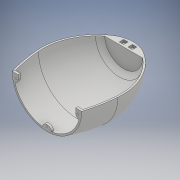
# Autodesk Inventor part: learnbotBack
Saved by Autodesk Inventor 2017 (Build 210142000, 142)
## iProperties
Part Number: learnbotBack
Material: Genérico
Document SubType Name: Modeling
Designer: rober
Density: 1 g/cm^3
Appearance: Valor por defecto
Author: rober
Autodesk Inventor part; units mm, degrees
ref_plane "YZ Plane" through (0, 0, 0) normal (1, 0, 0) x (0, 1, 0)
ref_plane "XZ Plane" through (0, 0, 0) normal (0, 1, 0) x (-1, 0, 0)
ref_plane "XY Plane" through (0, 0, 0) normal (0, 0, 1) x (1, 0, 0)
sketch "Boceto1" plane through (0, 0, 0) normal (0, 0, 1) x (1, 0, 0)
  arc A0 (-1.3629, 5.5333) -> (-0.3139, 0) centre (24.2256, 7.518) ccw
  arc A1 (-1.0638, 5.5565) -> (0, 0) centre (24.2256, 7.518) ccw
  arc A2 (3.3612, 14.9282) -> (1.4714, 13.4053) centre (8.9925, 6.0064) ccw
  arc A3 (3.5214, 14.6745) -> (1.6853, 13.1949) centre (8.9925, 6.0064) ccw
  arc A4 (6.03, 15.7) -> (3.3612, 14.9282) centre (6.03, 10.7) ccw
  arc A5 (6.03, 15.4) -> (3.5214, 14.6745) centre (6.03, 10.7) ccw
  arc A6 (1.4714, 13.4053) -> (-1.3629, 5.5333) centre (8.6002, 6.3924) ccw
  arc A7 (1.6853, 13.1949) -> (-1.0617, 5.5333) centre (8.6002, 6.3924) ccw
  line L0 (6.03, 15.4) -> (6.03, 15.7)
  line L1 (-0.3139, 0) -> (0, 0)
  line L2 (0, 0) -> (-0.3139, 0)
  line L3 (-1.0617, 5.5333) -> (-1.3629, 5.5333)
  arc A8 (-1.0617, 5.5333) -> (0, 0) centre (24.2008, 7.5121) ccw
  arc A9 (-1.3629, 5.5333) -> (-0.3139, 0) centre (24.2256, 7.518) ccw
  line L4 (6.03, 15.7) -> (6.03, 15.4)
  line L5 (4.6409, 15.5032) -> (4.7243, 15.215)
  arc A10 (6.03, 15.7) -> (4.6409, 15.5032) centre (6.03, 10.7) ccw
  arc A11 (6.03, 15.4) -> (4.7243, 15.215) centre (6.03, 10.7) ccw
  point P0 (0, 0)
  point P1 (0, 0)
  constraints: 26 point on circle, 12 centre point, 12 end point, 3 concentric, 1 collinear, 1 horizontal, 1 vertical
revolve "Revolución1" add sketch "Boceto1" angle 180 about axis through (6.03, 15.7, 0) along (0, -1, 0)
sketch "Boceto2" plane through (6.03, 0, 0) normal (0, -1, 0) x (1, 0, 0)
  line L0 (6.3439, 0) -> (5.2385, 0)
  line L1 (-6.3439, 0) -> (-5.2629, 0.0014)
  arc A0 (0.7982, -5.9748) -> (-0.7982, -5.9769) centre (0.0001, -6.0289) ccw
  arc A1 (5.2385, -0.7979) -> (5.8299, -1.5703) centre (6.0385, -0.7979) ccw
  line L2 (5.2385, -0.7979) -> (5.2385, 0)
  line L3 (-5.2629, 0.0014) -> (-5.2629, -0.7928)
  arc A2 (-5.822, -1.563) -> (-5.2629, -0.7928) centre (-6.0628, -0.8001) ccw
  line L4 (-0.7982, -5.9769) -> (-0.8064, -6.2925)
  arc A3 (-6.3439, 0) -> (6.3439, 0) centre (0, 0) ccw projected
  line L5 (0.7982, -5.9748) -> (0.79, -6.2925)
  line L6 (0.79, -6.2925) -> (-0.8064, -6.2925)
  line L7 (5.8299, -1.5703) -> (6.1465, -1.5703)
  line L8 (6.1465, -1.5703) -> (6.3439, 0)
  line L9 (-5.822, -1.563) -> (-6.1463, -1.563)
  line L10 (-6.1463, -1.563) -> (-6.3439, 0)
  line L11 (-6.3439, 0) -> (-6.03, 0) projected
  line L12 (6.03, 0) -> (6.3439, 0) projected
  point P0 (-6.03, 0)
  constraints: 22 end point, 7 point on circle, 3 centre point, 3 horizontal, 1 parallel
extrude "Extrusión1" add sketch "Boceto2" against normal blind 0.4 contours L8 L7 A1 L2 L0 | L10 L1 L3 A2 L9 | L4 A0 L5 L6
sketch "Boceto3" plane through (6.03, 10.7, 0) normal (0, 0, 1) x (1, 0, 0)
  arc A0 (-2.5086, 3.9745) -> (-4.3447, 2.4949) centre (2.9625, -4.6936) ccw projected
  arc A1 (2.5086, 3.9745) -> (-2.5086, 3.9745) centre (0, 0) ccw projected
  arc A2 (4.3447, 2.4949) -> (2.5086, 3.9745) centre (-2.9625, -4.6936) ccw projected
  line L0 (0, 4.7) -> (0, 3.3)
  line L1 (0, 3.3) -> (3.454, 3.3)
  arc A3 (2.5086, 3.9745) -> (0, 4.7) centre (0, 0) ccw
  arc A4 (3.454, 3.3) -> (2.5086, 3.9745) centre (-2.9625, -4.6936) ccw
  point P0 (-6.03, -10.7)
  dimension "d3" = 1.4
  constraints: 5 point on circle, 4 end point, 2 centre point, 2 concentric, 1 perpendicular, 1 vertical
  measures "d3" distance of L0.start L0.end
revolve "Revolución2" add sketch "Boceto3" angle 180 about axis through (6.03, 15.4, 0) along (0, 1, 0)
sketch "Boceto4" plane through (6.03, 10.7, 0) normal (0, 0, 1) x (1, 0, 0)
  line L0 (-3.454, 3.3) -> (3.454, 3.3) projected
  arc A0 (2.6688, 4.2282) -> (-2.6688, 4.2282) centre (0, 0) ccw projected
  line L1 (1.2, 3.7) -> (0.4, 3.7)
  line L2 (0.4, 3.7) -> (0.4, 4.5)
  line L3 (0.4, 4.5) -> (1.2, 4.5)
  line L4 (1.2, 4.5) -> (1.2, 3.7)
  line L5 (-1.2, 3.7) -> (-0.4, 3.7)
  line L6 (-0.4, 3.7) -> (-0.4, 4.5)
  line L7 (-0.4, 4.5) -> (-1.2, 4.5)
  line L8 (-1.2, 4.5) -> (-1.2, 3.7)
  point P0 (-6.03, -10.7)
  dimension "d11" = 0.8
  dimension "d12" = 0.8
  constraints: 16 end point, 1 horizontal, 1 perpendicular
  measures "d11" distance of L1.start L1.end
  measures "d12" distance of L1.end L2.end
extrude "Extrusión2" cut sketch "Boceto4" against normal blind 0.44
sketch "Boceto5" plane through (11.2684, 0, -0.7979) normal (0, -1, 0) x (1, 0, 0)
  arc A0 (-4.4402, -5.1769) -> (-6.0367, -5.179) centre (-5.2384, -5.231) ccw projected
  arc A1 (0, 0) -> (0.584, -0.7703) centre (0.8, 0) ccw projected
  arc A2 (-11.0604, -0.7651) -> (-10.5013, 0.0051) centre (-11.3013, -0.0022) ccw projected
  circle A3 centre (-5.239, -4.8045) radius 0.15
  circle A4 centre (-10.8572, 0.0051) radius 0.15
  line L0 (0, 0) -> (0, 0.7979) projected
  arc A5 (-4.4403, -5.179) -> (0.584, -0.7703) centre (-5.2385, 0.7979) ccw projected
  circle A6 centre (0.3733, 0) radius 0.15
  point P0 (-11.2684, 0.7979)
  dimension "d16" = 0.3
  dimension "d18" = 0.3
  constraints: 3 centre point
  measures "d16" diameter of A3
  measures "d18" diameter of A4
extrude "Extrusión3" cut sketch "Boceto5" against normal blind 0.8
